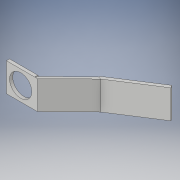
# Autodesk Inventor part: Spinner to Top
Saved by Autodesk Inventor 2017 (Build 210142000, 142)
## iProperties
Created: 2017-06-10
Part Number: Spinner to Top
Material: Generic
Document SubType Name: Modeling
Designer: Matthew
Density: 1 g/cm^3
Appearance: Default
Author: Matthew
Autodesk Inventor part; units mm, degrees
ref_plane "YZ Plane" through (0, 0, 0) normal (1, 0, 0) x (0, 1, 0)
ref_plane "XZ Plane" through (0, 0, 0) normal (0, 1, 0) x (-1, 0, 0)
ref_plane "XY Plane" through (0, 0, 0) normal (0, 0, 1) x (1, 0, 0)
sketch "Sketch1" plane through (0, 0, 0) normal (0, 1, 0) x (-1, 0, 0)
  line L0 (43.0137, 64.3915) -> (32.1817, 14.8739)
  line L1 (-10.5502, -12.5966) -> (-8.8333, -15.2673)
  line L2 (-8.8333, -15.2673) -> (35.0028, 12.913)
  line L3 (35.0028, 12.913) -> (46.1153, 63.713)
  line L4 (46.1153, 63.713) -> (43.0137, 64.3915)
  line L5 (-10.5502, -12.5966) -> (-10.5502, 12.913)
  line L6 (-10.5502, -12.5966) -> (32.1817, 14.8739)
  line L7 (46.1153, 63.713) -> (74.6903, 63.713)
  line L8 (74.6903, 63.713) -> (74.6903, 66.888)
  line L9 (74.6903, 66.888) -> (43.5598, 66.888)
  line L10 (43.0137, 64.3915) -> (43.5598, 66.888)
  point P0 (0, 0)
  dimension "d0" = 3.175
  dimension "d1" = 3.175
  dimension "d3" = 50.8
  dimension "d4" = 57.265
  dimension "d5" = 50.8
  dimension "d6" = 11.1125
  dimension "d7" = 28.575
  dimension "d8" = 3.175
  constraints: 22 end point, 4 perpendicular, 3 vertical, 1 collinear, 1 horizontal, 1 parallel, 1 other
  measures "d0" distance of L1.start L1.end
  measures "d1" distance of L3.end L0.start
  measures "d3" distance of L1.start L0.end
  measures "d4" angle of L5 L6
  measures "d5" vertical distance of L2.end L3.end
  measures "d6" horizontal distance of L2.end L3.end
  measures "d7" distance of L3.end L7.end
  measures "d8" distance of L7.end L8.end
extrude "Extrusion1" add sketch "Sketch1" along normal blind 28.575
sketch "Sketch2" plane through (-74.6903, 0, 66.888) normal (0, 0, 1) x (1, 0, 0)
  line L0 (28.575, 0) -> (0, 0) projected
  line L1 (0, 0) -> (0, 28.575) projected
  line L2 (28.575, 28.575) -> (0, 28.575) projected
  line L3 (28.575, 0) -> (28.575, 28.575) projected
  line L4 (28.575, 28.575) -> (0, 28.575) projected
  line L5 (0, 0) -> (0, 28.575) projected
  circle A0 centre (14.2875, 14.2875) radius 11.1125
  point P0 (74.6903, 0)
  point P1 (14.2875, 28.575)
  point P2 (0, 14.2875)
  dimension "d11" = 22.225
  constraints: 2 midpoint, 1 centre point
  measures "d11" diameter of A0
extrude "Extrusion2" cut sketch "Sketch2" against normal blind 28.575 contours A0
sketch "Sketch3" plane through (10.5502, 0, -12.5966) normal (0.5408, 0, 0.8412) x (0.8412, 0, -0.5408)
  line L0 (-50.8, 0) -> (-50.8, 28.575) projected
  line L1 (-50.8, 7.9375) -> (0, 7.9375)
  line L2 (0, 7.9375) -> (0, -20.6375)
  line L3 (0, -20.6375) -> (-50.8, -20.6375)
  line L4 (-50.8, -20.6375) -> (-50.8, 7.9375)
  line L5 (-50.8, 28.575) -> (0, 28.575) projected
  point P0 (-15.6863, 0)
  dimension "d14" = 50.8
  dimension "d15" = 28.575
  dimension "d16" = 20.6375
  constraints: 8 end point, 2 parallel, 1 horizontal, 1 perpendicular, 1 point on line
  measures "d14" distance of L2.end L3.end
  measures "d15" distance of L1.end L2.end
  measures "d16" distance from line of L5 L1.end
sketch "Sketch4" plane through (-32.1817, 0, 14.8739) normal (0.9769, 0, 0.2137) x (0.2137, 0, -0.9769)
  line L0 (-53.2441, 0) -> (-53.2441, 28.575) projected
  line L1 (-53.2441, 28.575) -> (0, 7.9375)
  line L2 (0, 0) -> (0, 28.575) projected
  line L3 (0, 7.9375) -> (0, -20.6375)
  line L4 (0, -20.6375) -> (-53.2441, 0)
  line L5 (-53.2441, 28.575) -> (-53.2441, 0)
  point P0 (21.4074, 0)
  dimension "d17" = 20.6375
  dimension "d18" = 28.575
  constraints: 8 end point, 1 collinear, 1 point on line, 1 vertical
  measures "d17" distance of L2.end L1.end
  measures "d18" distance of L1.end L3.end
sketch "Sketch5" plane through (-32.1817, 0, 14.8739) normal (0.9769, 0, 0.2137) x (0.2137, 0, -0.9769)
  line L0 (-53.2441, 41.9678) -> (42.8737, 41.9678)
  line L1 (42.8737, 41.9678) -> (42.8737, -28.4609)
  line L2 (42.8737, -28.4609) -> (-53.2441, -28.4609)
  line L3 (-53.2441, -28.4609) -> (-53.2441, 41.9678)
  point P0 (21.4074, 0)
  constraints: 8 end point, 2 parallel, 1 horizontal, 1 perpendicular
extrude "Extrusion3" cut sketch "Sketch5" along normal blind 50.8 and the other way blind 3.175
extrude "Extrusion4" add sketch "Sketch4" against normal blind 3.175
extrude "Extrusion5" add sketch "Sketch3" against normal blind 3.175
sketch "Sketch6" plane through (8.8333, 0, -15.2673) normal (-0.5408, 0, -0.8412) x (-0.8412, 0, 0.5408)
  line L0 (50.8, 7.9375) -> (0, 7.9375) projected
  line L1 (50.8, 7.9375) -> (63.8738, 7.9375)
  line L2 (63.8738, 7.9375) -> (63.8738, -20.6375)
  line L3 (63.8738, -20.6375) -> (50.8, -20.6375)
  line L4 (50.8, -20.6375) -> (50.8, 7.9375)
  point P0 (15.6863, 0)
  constraints: 8 end point, 2 parallel, 1 horizontal, 1 perpendicular
extrude "Extrusion6" add sketch "Sketch6" against normal blind 3.175
sketch "Sketch7" plane through (-35.2833, 0, 14.1954) normal (-0.9769, 0, -0.2137) x (-0.2137, 0, 0.9769)
  line L0 (50.6885, 27.5845) -> (0, 7.9375) projected
  line L1 (3.1832, -19.4037) -> (53.2441, 0) projected
  line L2 (0, 7.9375) -> (3.1832, 7.9375) projected
  line L3 (0, 7.9375) -> (-56.9759, -14.1465)
  line L4 (-56.9759, -14.1465) -> (-50.1301, -40.068)
  line L5 (53.2441, 0) -> (0, -20.6375) projected
  line L6 (-50.1301, -40.068) -> (0, -20.6375)
  line L7 (0, 7.9375) -> (-35.9676, 7.9375) projected
  line L8 (0, 7.9375) -> (0, -20.6375)
  line L9 (11.5155, 12.4009) -> (21.1446, -12.4418)
  line L10 (-34.1585, 31.8696) -> (27.6424, 31.8696)
  line L11 (27.6424, 31.8696) -> (27.6424, -37.0154)
  line L12 (27.6424, -37.0154) -> (-34.1585, -37.0154)
  line L13 (-34.1585, -37.0154) -> (-34.1585, 31.8696)
  point P0 (-21.4074, 0)
  constraints: 18 end point, 3 perpendicular, 2 collinear, 2 parallel, 2 point on line, 1 horizontal
extrude "Extrusion7" cut sketch "Sketch7" along normal blind 25.4 contours L9 L1 L5 L8 L0 | L0 L7 L13 L10 L11 | L0 L11 L1 L9 | L8 L6 L13 L3 | L3 L13 L7 | L1 L11 L12 L13 L6 L5
body "Solid1"
